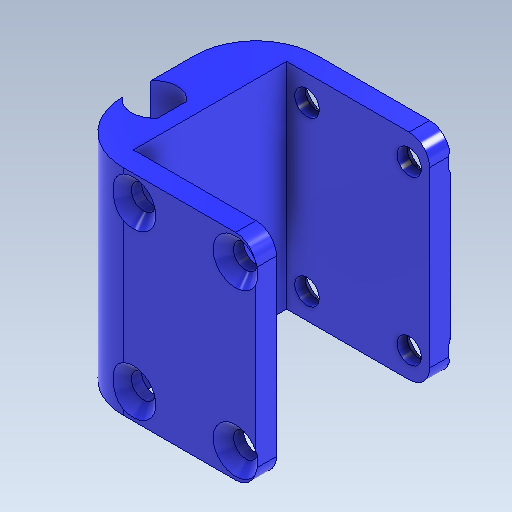
# Autodesk Inventor part: FINGERtopback panel
Saved by Autodesk Inventor 2020 (Build 240168000, 168)
## iProperties
Created: 2020-04-22
Part Number: FINGERtopback panel
Material: Generic
Document SubType Name: Modeling
Designer: sami_
Density: 1 g/cm^3
Appearance: Blue - Wall Paint - Glossy
Author: sami_
Autodesk Inventor part; units mm, degrees
ref_plane "YZ Plane" through (0, 0, 0) normal (1, 0, 0) x (0, 1, 0)
ref_plane "XZ Plane" through (0, 0, 0) normal (0, 1, 0) x (-1, 0, 0)
ref_plane "XY Plane" through (0, 0, 0) normal (0, 0, 1) x (1, 0, 0)
sketch "Sketch1" plane through (0, 0, 0) normal (0, 1, 0) x (-1, 0, 0)
  line L0 (0, 0) -> (14, 0)
  line L1 (14, 0) -> (14, -15)
  line L2 (14, -15) -> (0, -15)
  line L3 (0, -15) -> (0, 0)
  line L4 (0, 2) -> (19, 2)
  line L5 (19, 2) -> (19, -17)
  line L6 (19, -17) -> (0, -17)
  line L7 (0, -17) -> (0, 2)
  line L8 (19, 2) -> (14, 2) construction
  line L9 (14, 2) -> (14, -17) construction
  line L10 (14, -17) -> (19, -17) construction
  line L11 (19, -17) -> (19, 2) construction
  line L12 (15.5, 2) -> (15.5, -17)
  line L13 (15.5, 2) -> (19, -17) construction
  line L14 (19, 2) -> (15.5, -17) construction
  circle A0 centre (17.25, -5.3) radius 2.25
  line L15 (19, -3.8858) -> (19, -6.7142)
  line L16 (15.5, -3.8858) -> (15.5, -6.7142)
  line L17 (15.5, 2) -> (0, 2)
  line L18 (0, 2) -> (0, 6)
  line L19 (0, 6) -> (15.5, 6)
  line L20 (15.5, 6) -> (15.5, 2)
  line L21 (19, 2) -> (15.5, 2)
  line L22 (15.5, 2) -> (15.5, 6)
  line L23 (15.5, 6) -> (19, 6)
  line L24 (19, 6) -> (19, 2)
  point P0 (19, -6.7142)
  point P1 (19, -3.8858)
  point P2 (17.25, -7.5)
  dimension "d0" = 14
  dimension "d1" = 15
  dimension "d2" = 5
  dimension "d3" = 2
  dimension "d4" = 2
  dimension "d5" = 1.5
  dimension "d20" = 4.5
  dimension "d21" = 2.8284
  dimension "d47" = 5.3
  dimension "d49" = 4
  constraints: 50 end point, 10 parallel, 8 point on line, 6 perpendicular, 5 horizontal, 4 point on circle, 1 centre point, 1 midpoint, 1 vertical alignment
  measures "d0" distance of L1.end L2.end
  measures "d1" distance of L0.end L1.end
  measures "d2" distance between parallel lines of L1 L5
  measures "d3" distance between parallel lines of L0 L4
  measures "d4" distance between parallel lines of L6 L2
  measures "d5" distance between parallel lines of L1 L12
  measures "d20" diameter of A0
  measures "d21" distance of L15.start L15.end
  measures "d47" distance from line of L0 A0.centre
  measures "d49" distance of L17.end L18.end
extrude "Extrusion1" add sketch "Sketch1" along normal blind 21 contours L7 L4 L12 A0 L6 L2 L1 L0 | L4 L5 A0 L12 | L12 A0 L5 L6 | L12 A0
sketch "Sketch3" plane through (0, 0, -17) normal (0, 0, -1) x (-1, 0, 0)
  line L0 (19, 0) -> (19, 21) construction
  line L1 (15.5, 0) -> (15.5, 21) construction
  line L2 (19, 21) -> (15.5, 21) construction
  line L3 (15.5, 21) -> (15.5, 0) construction
  line L4 (15.5, 0) -> (19, 0) construction
  line L5 (19, 0) -> (19, 21) construction
  line L6 (19, 21) -> (15.5, 21) construction
  line L7 (15.5, 21) -> (15.5, 10.5) construction
  line L8 (15.5, 10.5) -> (19, 10.5) construction
  line L9 (19, 10.5) -> (19, 21) construction
  line L10 (19, 15.75) -> (15.5, 15.75) construction
  line L11 (15.5, 15.75) -> (15.5, 21) construction
  line L12 (15.5, 21) -> (19, 21) construction
  line L13 (19, 21) -> (19, 15.75) construction
  line L14 (19, 15.75) -> (17.5, 15.75)
  line L15 (17.5, 15.75) -> (17.5, 18.25)
  line L16 (17.5, 18.25) -> (19, 18.25)
  line L17 (19, 18.25) -> (19, 15.75)
  line L18 (17.5, 18.25) -> (15.5, 18.25)
  line L19 (15.5, 18.25) -> (15.5, 15.75)
  line L20 (15.5, 15.75) -> (17.5, 15.75)
  line L21 (17.5, 15.75) -> (17.5, 18.25)
  line L22 (19, 15.75) -> (15.5, 15.75)
  line L23 (15.5, 15.75) -> (15.5, 13.75)
  line L24 (15.5, 13.75) -> (19, 13.75)
  line L25 (19, 13.75) -> (19, 15.75)
  arc A0 (15.5, 15.75) -> (19, 13.75) centre (18.9642, 17.7498) ccw
  line L26 (19, 5.25) -> (15.5, 5.25) construction
  line L27 (19, 5.25) -> (17.5, 5.25)
  line L28 (17.5, 5.25) -> (17.5, 2.75)
  line L29 (17.5, 2.75) -> (19, 2.75)
  line L30 (19, 2.75) -> (19, 5.25)
  line L31 (17.5, 2.75) -> (15.5, 2.75)
  line L32 (15.5, 2.75) -> (15.5, 5.25)
  line L33 (15.5, 5.25) -> (17.5, 5.25)
  line L34 (17.5, 5.25) -> (17.5, 2.75)
  line L35 (19, 5.25) -> (15.5, 5.25)
  line L36 (15.5, 5.25) -> (15.5, 7.25)
  line L37 (15.5, 7.25) -> (19, 7.25)
  line L38 (19, 7.25) -> (19, 5.25)
  arc A1 (19, 7.25) -> (15.5, 5.25) centre (18.9642, 3.2502) ccw
  point P0 (0, 0)
  point P1 (18.9284, 13.75)
  point P2 (18.9284, 7.25)
  dimension "d11" = 1.5
  dimension "d12" = 2.5
  dimension "d13" = 2
  dimension "d14" = 4
  constraints: 74 end point, 12 parallel, 11 symmetric about line, 6 horizontal, 5 perpendicular, 4 point on circle, 2 centre point, 2 midpoint, 1 collinear, 1 other
  measures "d11" distance of L15.end L16.end
  measures "d12" distance of L14.end L15.end
  measures "d13" distance of L23.end L22.end
  measures "d14" radius of A0
extrude "Extrusion2" cut sketch "Sketch3" against normal up to surface contours L27 L33 A1 L38 | L28 L31 L32 L33
fillet "Fillet2" radius 1 3 edges at (-15.5, 5.25, -11.8571) (-15.5, 2.75, -11.8571) (-17.5, 2.75, -12.268)
sketch "Sketch4" plane through (0, 0, -17) normal (0, 0, -1) x (-1, 0, 0)
  line L0 (0, 21) -> (19, 21) projected
  line L1 (14, 0) -> (14, 21) projected
  line L2 (0, 21) -> (14, 21)
  line L3 (14, 21) -> (14, 0)
  line L4 (14, 0) -> (0, 0)
  line L5 (0, 0) -> (0, 21)
  circle A0 centre (12, 18.5) radius 1
  circle A1 centre (12, 2.5) radius 1
  circle A2 centre (2, 18.5) radius 1
  circle A3 centre (2, 2.5) radius 1
  line L6 (12, 18.5) -> (2, 18.5)
  line L7 (2, 18.5) -> (2, 2.5)
  line L8 (2, 2.5) -> (12, 2.5)
  line L9 (12, 2.5) -> (12, 18.5)
  point P0 (0, 0)
  dimension "d22" = 2
  dimension "d23" = 2
  dimension "d24" = 2
  dimension "d25" = 2
  dimension "d26" = 10
  dimension "d27" = 16
  dimension "d28" = 2.5
  dimension "d29" = 2.5
  dimension "d30" = 2
  dimension "d31" = 2
  constraints: 16 end point, 4 centre point, 4 coincident, 4 parallel, 2 horizontal, 2 perpendicular
  measures "d22" diameter of A0
  measures "d23" diameter of A1
  measures "d24" diameter of A2
  measures "d25" diameter of A3
  measures "d26" distance of L8.end L7.end
  measures "d27" distance of L7.end L6.end
  measures "d28" distance between parallel lines of L4 L8
  measures "d29" distance between parallel lines of L0 L6
  measures "d30" distance between parallel lines of L1 L9
  measures "d31" distance between parallel lines of L5 L7
hole "Hole1" at (-12, 18.5, -17) at (-12, 2.5, -17) at (-2, 2.5, -17) at (-2, 18.5, -17) direction (0, 0, 1) diameter 2.4 end through all countersink diameter 4.4 countersink angle 90 clearance for "Countersunk Flat Head Screw ISO 2009/7046" size "M2" standard "ISO"
sketch "Sketch5" plane through (-19, 0, 2) normal (0, 0, 1) x (1, 0, 0)
  circle A0 centre (7, 2.5) radius 1.2 projected
  circle A1 centre (7, 2.5) radius 0.7835
  circle A2 centre (7, 18.5) radius 1.2 projected
  circle A3 centre (7, 18.5) radius 0.7835
  circle A4 centre (17, 18.5) radius 1.2 projected
  circle A5 centre (17, 18.5) radius 0.7835
  circle A6 centre (17, 2.5) radius 1.2 projected
  circle A7 centre (17, 2.5) radius 0.7835
  point P0 (19, 0)
  constraints: 4 centre point, 4 coincident
hole "Hole2" at (-12, 18.5, 2) at (-12, 2.5, 2) at (-2, 2.5, 2) at (-2, 18.5, 2) direction (0, 0, -1) diameter 2.4 end through all countersink diameter 4.4 countersink angle 90 clearance for "Countersunk Flat Head Screw ISO 2009/7046" size "M2" standard "ISO"
fillet "Fillet5" radius 6 3 edges at (-19, 10.5, 2) (-19, 2.625, -17) (-19, 14.125, -17)
fillet "Fillet6" radius 2 4 edges at (0, 0, 1) (0, 0, -16) (0, 21, -16) (0, 21, 1)
equation "\"d4\" = d3"
equation "\"d28\" = d29"
equation "\"d30\" = d31"
body "Solid1"
